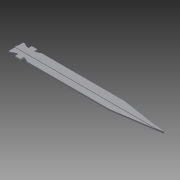
# Autodesk Inventor part: Hoja
Saved by Autodesk Inventor 2011 (Build 150239000, 239)
## iProperties
Created: 2014-08-04
Part Number: Hoja
Material: Por defecto
Document SubType Name: Chapa
Designer: amatiasq
Density: 1 g/cm^3
Sheet Metal Rule: Por defecto_mm
Author: amatiasq
Autodesk Inventor part; units mm, degrees
ref_plane "YZ Plane" through (0, 0, 0) normal (1, 0, 0) x (0, 1, 0)
ref_plane "XZ Plane" through (0, 0, 0) normal (0, 1, 0) x (-1, 0, 0)
ref_plane "XY Plane" through (0, 0, 0) normal (0, 0, 1) x (1, 0, 0)
sketch "Boceto1" plane through (0, 0, 0) normal (0, 0, 1) x (1, 0, 0)
  line L0 (0, 0) -> (0, -10.8)
  line L1 (0, -10.8) -> (3, -10.8)
  arc A0 (11, -7.6) -> (3, -10.8) centre (11.1596, -19.5989) ccw
  line L2 (11, -7.6) -> (11, -12.6)
  line L3 (11, -12.6) -> (19, -12.6)
  line L4 (19, -12.6) -> (19, -7.6)
  arc A1 (27, -10.8) -> (19, -7.6) centre (18.8404, -19.5989) ccw
  line L5 (27, -10.8) -> (150, -10.8)
  line L6 (220, 0) -> (150, -10.8)
  line L7 (0, 0) -> (0, 10.8)
  line L8 (0, 10.8) -> (3, 10.8)
  arc A2 (3, 10.8) -> (11, 7.6) centre (11.1596, 19.5989) ccw
  line L9 (11, 7.6) -> (11, 12.6)
  line L10 (11, 12.6) -> (19, 12.6)
  line L11 (19, 12.6) -> (19, 7.6)
  arc A3 (19, 7.6) -> (27, 10.8) centre (18.8404, 19.5989) ccw
  line L12 (27, 10.8) -> (150, 10.8)
  line L13 (220, 0) -> (150, 10.8)
  dimension "d0" = 10.8
  dimension "d1" = 3
  dimension "d2" = 12
  dimension "d3" = 5
  dimension "d4" = 8
  dimension "d5" = 5
  dimension "d6" = 12
  dimension "d7" = 123
  constraints: 28 end point, 8 point on circle, 4 centre point, 4 perpendicular, 1 parallel, 1 vertical
  measures "d0" distance of L0.start L0.end
  measures "d1" distance of L0.end L1.end
  measures "d2" radius of A0
  measures "d3" distance of L2.start L2.end
  measures "d4" distance of L2.end L3.end
  measures "d5" distance of L3.end L4.end
  measures "d6" radius of A1
  measures "d7" distance of L5.start L5.end
extrude "Extrusión1" add sketch "Boceto1" along normal blind 2
sketch "Boceto2" plane through (0, 0, 2) normal (0, 0, 1) x (1, 0, 0)
  line L0 (0, -10.8) -> (0, 10.8) projected
  line L1 (220, 0) -> (150, -10.8) projected
  line L2 (150, 10.8) -> (220, 0) projected
  line L3 (0, 10.8) -> (3, 10.8) projected
  line L4 (0, -1.7) -> (208.9815, -1.7)
  line L5 (0, 1.7) -> (208.9815, 1.7)
  point P0 (0, 0)
  constraints: 4 end point, 4 point on line, 2 parallel
extrude "Extrusión2" add sketch "Boceto2" along normal blind 0.7
equation "\"Radio_pliegue\" = Grosor"
equation "\"Anchura_desahogo_plegado\" = Grosor"
equation "\"Profundidad_desahogo_plegado\" = 0.5 * Grosor"
equation "\"Tamaño_destalonado\" = 4 * Grosor"
equation "\"Remanente_mínimo\" = 2 * Grosor"
equation "\"Radiodetransición\" = Radio_pliegue"
equation "\"Tamaño_de_radio_de_Jacobi\" = Radio_pliegue"
equation "\"TamañoSeparación\" = Grosor"
equation "\"Grosor\" = 0.5"
